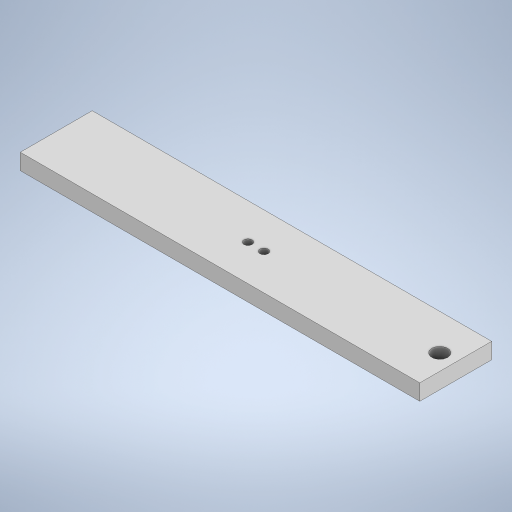
# Autodesk Inventor part: 다리-3
Saved by Autodesk Inventor 2024 (Build 280153000, 153)
## iProperties
Created: 2024-09-10
Part Number: 다리-3
Material: 일반
Document SubType Name: Modeling
Designer: USER
Density: 1 g/cm^3
Appearance: 기본값
Author: USER
Autodesk Inventor part; units mm, degrees
sketch "스케치1" plane through (0, 0, 0) normal (0, 0, 1) x (1, 0, 0)
  line L0 (0, 0) -> (250, 0)
  line L1 (250, 0) -> (250, 10)
  line L2 (250, 10) -> (0, 10)
  line L3 (0, 10) -> (0, 0)
  dimension "d0" = 250
  dimension "d1" = 10
  constraints: 8 end point, 2 parallel, 1 horizontal, 1 perpendicular
  measures "d0" distance of L1.end L2.end
  measures "d1" distance between parallel lines of L0 L2
extrude "돌출1" add sketch "스케치1" along normal blind 45
ref_plane "작업 평면1" through (125, 0, 0) normal (-1, 0, 0) x (0, 0, 1)
ref_plane "작업 평면2" through (65, 40, 45) normal (0, 1, 0) x (1, 0, 0)
ref_plane "작업 평면3" through (125, 0, 0) normal (1, 0, 0) x (0, 0, -1)
sketch "스케치4" plane through (0, 10, 0) normal (0, 1, 0) x (1, 0, 0)
  line L0 (250, 0) -> (0, 0) projected
  line L1 (0, 0) -> (0, -45) projected
  line L2 (250, -45) -> (0, -45) projected
  line L3 (250, 0) -> (250, -45) projected
  circle A0 centre (120, -22.5) radius 2.6
  circle A1 centre (130, -22.5) radius 2.6
  line L4 (250, 0) -> (0, 0) projected
  point P0 (125, 0)
  point P1 (125, 0)
  dimension "d16" = 5.2
  dimension "d17" = 5.2
  dimension "d18" = 10
  dimension "d19" = 5
  constraints: 2 centre point, 2 midpoint, 1 horizontal alignment
  measures "d16" diameter of A1
  measures "d17" diameter of A0
  measures "d18" distance of A1.centre A0.centre
  measures "d19" horizontal distance of A0.centre point (125, 0)
extrude "돌출4" cut sketch "스케치4" against normal through all contours A0 | A1
ref_plane "작업 평면4" through (0, 0, 22.5) normal (0, 0, -1) x (-1, 0, 0)
sketch "스케치6" plane through (0, 10, 0) normal (0, 1, 0) x (1, 0, 0)
  line L0 (250, 0) -> (250, -45) projected
  circle A0 centre (240, -22.5) radius 5
  point P0 (0, 0)
  point P1 (250, -22.5)
  point P2 (250, -22.5)
  dimension "d32" = 10
  dimension "d33" = 10
  constraints: 2 midpoint, 1 centre point, 1 horizontal alignment
  measures "d32" diameter of A0
  measures "d33" distance from line of L0 A0.centre
extrude "돌출6" cut sketch "스케치6" against normal through all
